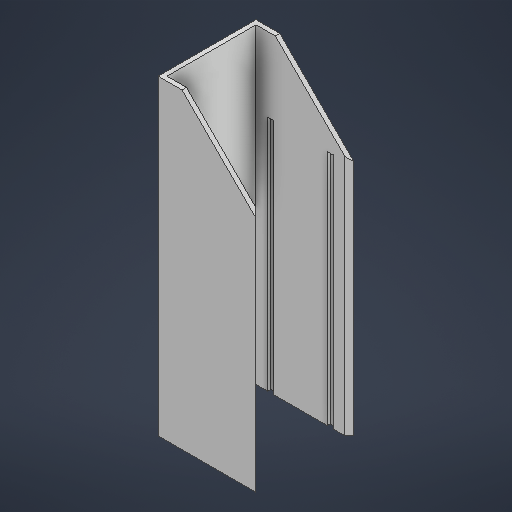
# Autodesk Inventor part: Frame
Saved by Autodesk Inventor 2027 (Build 310192060, 192F)
## iProperties
Created: 2026-07-05
Part Number: Frame
Material: Ogólny
Document SubType Name: Modeling
Designer: User
Density: 1 g/cm^3
Appearance: Domyślna
Author: User
Autodesk Inventor part; units mm, degrees
ref_plane "YZ Plane" through (0, 0, 0) normal (1, 0, 0) x (0, 1, 0)
ref_plane "XZ Plane" through (0, 0, 0) normal (0, 1, 0) x (-1, 0, 0)
ref_plane "XY Plane" through (0, 0, 0) normal (0, 0, 1) x (1, 0, 0)
sketch "Szkic1" plane through (0, 0, 0) normal (0, 1, 0) x (-1, 0, 0)
  line L0 (-16.5, 16.5) -> (16.5, 16.5)
  line L1 (16.5, 16.5) -> (16.5, -16.5)
  line L2 (16.5, -16.5) -> (-16.5, -16.5)
  line L3 (-16.5, -16.5) -> (-16.5, 16.5)
  line L4 (-16.5, 16.5) -> (16.5, -16.5) construction
  line L5 (16.5, 16.5) -> (-16.5, -16.5) construction
  line L6 (-15, -15) -> (15, -15)
  line L7 (15, -15) -> (15, 15)
  line L8 (15, 15) -> (-15, 15)
  line L9 (-15, 15) -> (-15, -15)
  line L10 (-15, -15) -> (15, 15) construction
  line L11 (15, -15) -> (-15, 15) construction
  line L12 (15, 15) -> (11, 15)
  line L13 (11, 15) -> (11, 16)
  line L14 (11, 16) -> (9, 16)
  line L15 (9, 16) -> (9, 15)
  line L16 (-15, 15) -> (-16.5, 16.5)
  line L17 (-15, -15) -> (-16.5, -16.5)
  line L18 (-9, 16) -> (-11, 16)
  line L19 (-11, 16) -> (-11, 15)
  line L20 (-9, 15) -> (-9, 16)
  line L21 (15, 0) -> (-15, 0) construction
  line L22 (11, -15) -> (11, -16)
  line L23 (11, -16) -> (9, -16)
  line L24 (9, -16) -> (9, -15)
  line L25 (-9, -16) -> (-11, -16)
  line L26 (-11, -16) -> (-11, -15)
  line L27 (-9, -15) -> (-9, -16)
  point P0 (0, 0)
  dimension "d0" = 33
  dimension "d1" = 33
  dimension "d2" = 30
  dimension "d3" = 30
  dimension "d4" = 4
  dimension "d5" = 1
  dimension "d6" = 2
  dimension "d7" = 1
  dimension "d10" = 20
  constraints: 56 end point, 8 symmetric about line, 6 midpoint, 4 parallel, 3 horizontal, 3 perpendicular, 2 point on line, 1 vertical, 7 other
  measures "d0" distance of L1.end L2.end
  measures "d1" distance of L0.end L1.end
  measures "d2" distance of L8.end L7.end
  measures "d3" distance of L7.end L6.end
  measures "d4" distance of L7.end L12.end
  measures "d5" distance of L12.end L13.end
  measures "d6" distance of L13.end L14.end
  measures "d7" distance of L14.end L15.end
  measures "d10" distance of L14.end L18.end
extrude "Wyciągnięcie proste1" add sketch "Szkic1" along normal blind 80 contours L0 L1 L2 L17 L6 L26 L25 L27 L24 L23 L22 L7 L8 L13 L14 L15 L20 L18 L19 L16
sketch "Szkic2" plane through (0, 80, 0) normal (0, 1, 0) x (1, 0, 0)
  line L0 (-16.5, 16.5) -> (-16.5, -16.5) projected
  line L1 (16.5, 16.5) -> (-16.5, 16.5)
  line L2 (-16.5, 16.5) -> (-16.5, -16.5)
  line L3 (-16.5, -16.5) -> (16.5, -16.5)
  line L4 (16.5, -16.5) -> (16.5, 16.5)
  line L5 (16.5, 16.5) -> (-16.5, -16.5) construction
  line L6 (-16.5, 16.5) -> (16.5, -16.5) construction
  line L7 (15, 15) -> (-15, 15)
  line L8 (-15, 15) -> (-15, -15)
  line L9 (-15, -15) -> (15, -15)
  line L10 (15, -15) -> (15, 15)
  line L11 (15, 15) -> (-15, -15) construction
  line L12 (-15, 15) -> (15, -15) construction
  line L13 (15, -15) -> (16.5, -16.5)
  line L14 (15, 15) -> (16.5, 16.5)
  point P0 (0, 0)
  dimension "d17" = 30
  constraints: 28 end point, 4 midpoint, 4 parallel, 3 perpendicular, 2 horizontal, 1 collinear, 1 point on line
  measures "d17" distance of L7.start L7.end
ref_plane "Płaszczyzna konstrukcyjna2" through (0.7685, 95.7685, 15) normal (0.7071068, 0.7071068, 0) x (0, 0, -1)
ref_plane "Płaszczyzna konstrukcyjna1" through (-15, 80, 15) normal (0.7071068, 0.7071068, 0) x (0, 0, -1)
extrude "Wyciągnięcie proste2" add sketch "Szkic2" along normal blind 25 contours L1 L14 L7 L8 L9 L13 L3 L0
sketch "Szkic3" plane through (0.7685, 95.7685, 15) normal (0.7071068, 0.7071068, 0) x (0, 0, -1)
  line L0 (-27.5895, -45.177) -> (54.5421, -45.177)
  line L1 (54.5421, -45.177) -> (54.5421, 37.234)
  line L2 (54.5421, 37.234) -> (-27.5895, 37.234)
  line L3 (-27.5895, 37.234) -> (-27.5895, -45.177)
  line L4 (-27.5895, -45.177) -> (54.5421, 37.234) construction
  line L5 (54.5421, -45.177) -> (-27.5895, 37.234) construction
  point P0 (15, -67.1751)
  point P1 (13.4763, -3.9715)
  constraints: 12 end point, 2 midpoint, 2 parallel, 1 horizontal, 1 perpendicular
extrude "Wyciągnięcie proste3" cut sketch "Szkic3" along normal blind 25
